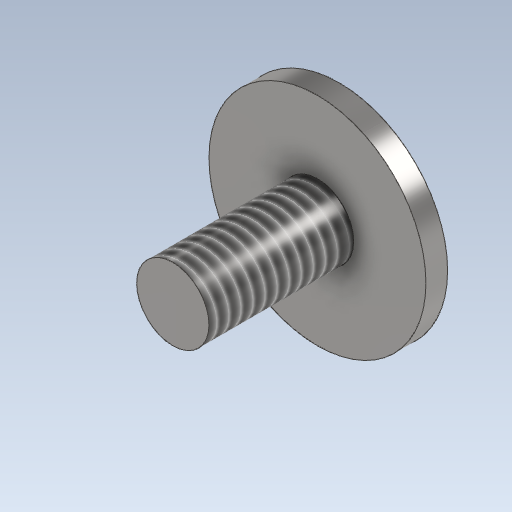
# Autodesk Inventor part: FreeHorn_Screw
Saved by Autodesk Inventor 2020.4 (Build 244396000, 396)
## iProperties
Part Number: FreeHorn_Screw
Material: ステンレス鋼 AISI 304
Document SubType Name: Modeling
Designer: Masato Kubotera
Density: 8 g/cm^3
Appearance: 半つや出し
Catalog Web Link: https://kondo-robot.com/product/02137
Description: ReadyMade
Author: Masato Kubotera
Autodesk Inventor part; units mm, degrees
ref_plane "YZ Plane" through (0, 0, 0) normal (1, 0, 0) x (0, 1, 0)
ref_plane "XZ Plane" through (0, 0, 0) normal (0, 1, 0) x (-1, 0, 0)
ref_plane "XY Plane" through (0, 0, 0) normal (0, 0, 1) x (1, 0, 0)
sketch "スケッチ1" plane through (0, 0, 0) normal (0, 1, 0) x (-1, 0, 0)
  line L0 (0, 0) -> (-4.5, 0)
  line L1 (-4.5, 0) -> (-4.5, 0.9)
  line L2 (-4.5, 0.9) -> (-1.5, 0.9)
  line L3 (-1.5, 0.9) -> (-1.5, 6.9)
  line L4 (-1.5, 6.9) -> (0, 6.9)
  line L5 (0, 6.9) -> (0, 0)
  dimension "d0" = 6
  dimension "d1" = 0.9
  dimension "d2" = 9
  dimension "d3" = 3
  constraints: 12 end point, 5 perpendicular, 1 horizontal
  measures "d0" distance of L2.end L3.end
  measures "d1" distance of L0.end L1.end
  measures "d2" diameter of L0.end L5
  measures "d3" diameter of L3.end L5
revolve "回転1" add sketch "スケッチ1" angle 360 about axis through (0, 0, 6.9) along (0, 0, -1)
thread "ねじ1" size "M3x0.5" class "6g" standard "ANSI Metric M Profile" length 7.57
